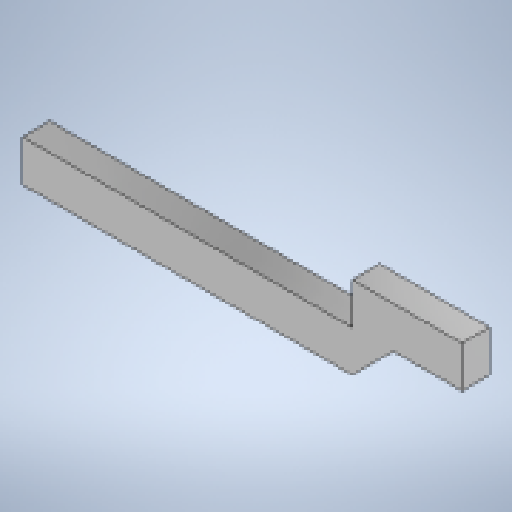
# Autodesk Inventor part: Teeth
Saved by Autodesk Inventor 2023.2 (Build 272271000, 271)
## iProperties
Created: 2024-01-16
Part Number: Teeth
Material: Aluminum 6061
Document SubType Name: Modeling
Designer: Nathan Cai
Density: 2.7 g/cm^3
Appearance: Aluminum - Flat
Author: Nathan Cai
Autodesk Inventor part; units mm, degrees
ref_plane "YZ Plane" through (0, 0, 0) normal (1, 0, 0) x (0, 1, 0)
ref_plane "XZ Plane" through (0, 0, 0) normal (0, 1, 0) x (-1, 0, 0)
ref_plane "XY Plane" through (0, 0, 0) normal (0, 0, 1) x (1, 0, 0)
sketch "Sketch1" plane through (0, 0, 0) normal (0, 0, 1) x (1, 0, 0)
  line L0 (-50.8, -4.7625) -> (50.8, -4.7625)
  line L1 (50.8, -4.7625) -> (50.8, 4.7625)
  line L2 (50.8, 4.7625) -> (-50.8, 4.7625)
  line L3 (-50.8, 4.7625) -> (-50.8, -4.7625)
  line L4 (-50.8, -4.7625) -> (50.8, 4.7625) construction
  line L5 (50.8, -4.7625) -> (-50.8, 4.7625) construction
  line L6 (50.8, 4.7625) -> (25.4, 4.7625)
  line L7 (25.4, 4.7625) -> (25.4, 14.2875)
  line L8 (25.4, 14.2875) -> (50.8, 14.2875)
  line L9 (50.8, 14.2875) -> (50.8, 4.7625)
  line L10 (25.4, -4.7625) -> (34.925, 4.7625)
  point P0 (0, 0)
  dimension "d0" = 101.6
  dimension "d1" = 9.525
  dimension "d2" = 25.4
  dimension "d3" = 9.525
  dimension "d4" = 45
  constraints: 22 end point, 4 parallel, 3 point on line, 2 horizontal, 2 midpoint, 2 perpendicular
  measures "d0" distance of L2.end L1.end
  measures "d1" distance of L1.end L0.end
  measures "d2" distance of L7.end L8.end
  measures "d3" distance of L6.end L7.end
  measures "d4" angle of L0 L10
extrude "Extrusion1" add sketch "Sketch1" along normal blind 6.35 contours L3 L2 L10 L0 | L2 L7 L8 L9
fillet "Fillet1" radius 3.175 3 edges at (25.4, 4.7625, 3.175) (34.925, 4.7625, 3.175) (25.4, -4.7625, 3.175)
chamfer "Chamfer1" distance 3.175 angle 45 2 edges at (25.4, 14.2875, 3.175) (-50.8, -4.7625, 3.175)
body "Solid1"
